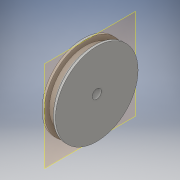
# Autodesk Inventor part: Wheel
Saved by Autodesk Inventor 2016 SP1 (Build 200210100, 210)
## iProperties
Created: 2016-02-06
Part Number: Wheel
Material: Generic
Document SubType Name: Modeling
Designer: steele
Density: 1 g/cm^3
Appearance: Default
Author: steele
Autodesk Inventor part; units mm, degrees
ref_plane "XZ Plane" through (0, 0, 0) normal (0, 1, 0) x (-1, 0, 0)
ref_plane "XY Plane" through (0, 0, 0) normal (0, 0, 1) x (1, 0, 0)
sketch "Sketch1" plane through (0, 0, 0) normal (1, 0, 0) x (0, 1, 0)
  circle A0 centre (0, 0) radius 101.6
  circle A1 centre (0, 0) radius 12.7
  dimension "d0" = 203.2
  dimension "d1" = 25.4
  constraints: 2 centre point, 2 coincident
  measures "d0" diameter of A0
  measures "d1" diameter of A1
extrude "Extrusion1" add sketch "Sketch1" along normal mid plane 25.4
sketch "Sketch3" plane through (12.7, 0, 0) normal (1, 0, 0) x (0, 0, -1)
  circle A0 centre (0, 0) radius 12.7
  circle A1 centre (0, 0) radius 115.8875
  dimension "d7" = 25.4
  dimension "d8" = 231.775
  constraints: 2 centre point, 2 coincident
  measures "d7" diameter of A0
  measures "d8" diameter of A1
extrude "Extrusion3" add sketch "Sketch3" along normal blind 6.35
mirror "Mirror1" about plane through (0, 0, 0) normal (1, 0, 0) of "Extrusion3"
body "Solid1"
